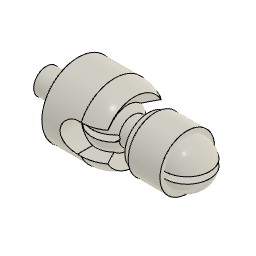
BallJoint2nd v2 (Autodesk Fusion 360 design; units mm, degrees)
Autodesk Fusion 360 part; units mm, degrees
sketch "スケッチ1" plane through (0, 0, 0) normal (0, 1, 0) x (1, 0, 0) in component "はめ込みジョイント"
  circle A0 centre (0, 0) radius 2.5
  line L0 (10, 1.5) -> (-2, 1.5)
  line L1 (-2, -1.5) -> (10, -1.5)
  line L2 (10, -1.5) -> (10, 1.5)
  line L3 (-2.5, 0) -> (10, 0)
  line L4 (1.7701, -0.35) -> (-2.4754, -0.35)
  line L5 (1.7701, 0.35) -> (-2.4754, 0.35)
  arc A1 (1.7701, -0.35) -> (1.7701, 0.35) centre (1.7701, 0) ccw
  dimension "d1" = 5
  dimension "d4" = 0.7
  constraint horizontal L0
  constraint parallel L0 L1
  constraint coincident A0.centre origin
  constraint midpoint L2 L3.end
  constraint coincident A0 L1.start
  constraint coincident A0 L3.start
  constraint coincident A0 L0.end
  constraint coincident L3 A1.centre
  constraint coincident A0 L4.end
  constraint tangent L4 A1
  constraint tangent L5 A1
  measures "d1" diameter of A0
  measures "d4" diameter of A1
revolve "回転1" add sketch "スケッチ1" angle 360 about axis through (-2.5, 0, 0) along (1, 0, 0) contours A0 L3 L4 A1 | A0 L1 L2 L3 | A0 L1 L3 L4 A1 | A0 L1 makes body 1 in component "はめ込みジョイント"
extrude "押し出し1" cut sketch "スケッチ1" along normal mid plane 6.2 contours A0 L3 L5 A1 | A0 L3 L4 A1 bodies 1 in component "はめ込みジョイント"
move_face "面を移動1" by (-6, 0, 0) 1 faces at (10, 0.5633, 0.8262) on bodies 1 in component "はめ込みジョイント"
mirror "ミラー1" about plane through (4, 0, 0) normal (1, 0, 0) of bodies 1 merged in component "はめ込みジョイント"
copy_body "ボディのコピーと貼り付け1" bodies 1 makes body 2 in component "はめ込みジョイント"
ref_plane "作業平面1" through (3, 0, 0) normal (1, 0, 0) x (0, 1, 0) in component "はめ込みジョイント"
split "分割1" by plane through (3, 0, 0) normal (1, 0, 0) bodies 2 makes body 3 at (7.9739, 2.1321, -1.3051) in component "はめ込みジョイント"
delete_body "RemoveBody1" bodies 3 in component "はめ込みジョイント"
ref_plane "作業平面2" through (4, 0, 0) normal (1, 0, 0) x (0, 1, 0) in component "はめ込みジョイント"
sketch "スケッチ2" plane through (4, 0, 0) normal (1, 0, 0) x (0, 1, 0) in component "はめ込みジョイント"
  circle A0 centre (0, 0) radius 3
  dimension "d12" = 6
  constraint coincident A0.centre origin
  measures "d12" diameter of A0
loft "ロフト1" add profiles "スケッチ2" section 1 face at (3, 0.5633, 0.8262) section 2 on bodies 2 bodies 2 in component "はめ込みジョイント"
extrude "押し出し2" add 1 faces at (4, -0.4661, 1.6472) along direction (1, 0, 0) blind 3 on bodies 2 bodies 2 in component "はめ込みジョイント"
sketch "スケッチ3" plane through (7, 0, 0) normal (1, 0, 0) x (0, 1, 0) in component "はめ込みジョイント"
  circle A0 centre (0, 0) radius 3
  circle A1 centre (0, 0) radius 1.6
  dimension "d15" = 3.2
  constraint concentric A0 A1
  measures "d15" diameter of A1
extrude "押し出し3" cut sketch "スケッチ3" against normal blind 3 contours A1 bodies 2 in component "はめ込みジョイント"
chamfer "面取り1" distance 0.5 angle 45 1 edges at (4, -2.797, 1.0848) on bodies 2 in component "はめ込みジョイント"
move_face "面を移動2" by (1, 0, 0) 1 faces at (7, -0.1889, 2.5207) on bodies 2 in component "はめ込みジョイント"
sketch "スケッチ4" plane through (0, 0, 0) normal (0, 1, 0) x (1, 0, 0) in component "はめ込みジョイント"
  circle A0 centre (0, 0) radius 2.6
  circle A1 centre (0, 0) radius 4
  line L0 (0, 0) -> (3, 0)
  line L1 (0, 0) -> (2.2021, -3.3393)
  line L2 (0, 0) -> (2.2021, 3.3393)
  line L3 (0, 0) -> (0, -0.2614)
  line L4 (0, -0.2614) -> (0, -4)
  line L5 (0, -4) -> (-4, -4)
  line L6 (-4, -4) -> (-4, 0)
  line L7 (-4, -4) -> (-8, -4)
  line L8 (-8, -4) -> (-8, 4)
  line L9 (-8, 4) -> (0, 4)
  line L10 (0, 0) -> (-8, 0)
  dimension "d19" = 5.2
  constraint coincident A0.centre A1.centre
  constraint coincident A1 L1.end
  constraint symmetric L0 A0.centre A1.centre
  constraint symmetric L0 L1.end L2.end
  constraint perpendicular L0 L3
  constraint coincident A1 L4.end
  constraint parallel L3 L4
  constraint tangent A1 L5
  constraint coincident A1 L6.end
  constraint tangent A1 L6
  constraint perpendicular L5 L6
  constraint perpendicular L6 L7
  constraint perpendicular L5 L8
  constraint coincident A1 L9.end
  constraint tangent A1 L9
  constraint perpendicular L8 L9
  constraint midpoint L8 L10.end
  measures "d19" diameter of A0
revolve "回転2" add sketch "スケッチ4" angle 360 about axis through (0, 0, 0) along (-1, 0, 0) separate body contours A0 A1 L1 L4 | A0 A1 L4 L10 | A1 L5 L6 | L6 L7 L8 L10 makes body 4 in component "はめ込みジョイント"
sketch "スケッチ5" plane through (0, 0, 0) normal (0, 1, 0) x (1, 0, 0) in component "はめ込みジョイント"
  circle A0 centre (-0.4, 0) radius 1.6
  line L0 (-0.4, 0) -> (-0.4, -1.6)
  line L1 (-0.4, 0) -> (-0.4, 1.6)
  line L2 (-0.4, -1.6) -> (4.9, -1.6)
  line L3 (4.9, -1.6) -> (4.9, 1.6)
  line L4 (4.9, 1.6) -> (-0.4, 1.6)
  dimension "d22" = 3.2
  constraint coincident A0.centre L0.start
  constraint vertical L0
  constraint coincident A0 L1.end
  constraint parallel L0 L1
  constraint perpendicular L0 L2
  constraint perpendicular L2 L3
  constraint perpendicular L1 L4
  measures "d22" diameter of A0
extrude "押し出し4" cut sketch "スケッチ5" along normal mid plane 9.2 bodies 4 in component "はめ込みジョイント"
sketch "スケッチ6" plane through (-8, 0, 0) normal (-1, 0, 0) x (0, -1, 0) in component "はめ込みジョイント"
  circle A0 centre (0, 0) radius 4
  circle A1 centre (0, 0) radius 1.6
  dimension "d25" = 3.2
  constraint coincident A0.centre A1.centre
  measures "d25" diameter of A1
extrude "押し出し5" cut sketch "スケッチ6" against normal blind 4 contours A1 bodies 4 in component "はめ込みジョイント"
copy_body "ボディのコピーと貼り付け2" bodies 4 makes body 5 in component "はめ込みジョイント"
extrude "押し出し6" cut 1 faces at (-8, -0.2386, 3.1836) along direction (1, 0, 0) blind 4 on bodies 5 bodies 5 in component "はめ込みジョイント"
move_face "面を移動3" by (0.5, 0, 0) 1 faces at (-4, 0.1832, -0.5939) on bodies 5 in component "はめ込みジョイント"
move_face "面を移動4" by (-0.5, 0, 0) 1 faces at (-3.5, 0.1832, -0.5939) on bodies 5 in component "はめ込みジョイント"
sketch "スケッチ7" plane through (-4, 0, 0) normal (-1, 0, 0) x (0, -1, 0) in component "はめ込みジョイント"
  circle A0 centre (0, 0) radius 4
  circle A1 centre (0, 0) radius 1.4
  dimension "d30" = 2.8
  constraint coincident A0.centre A1.centre
  measures "d30" diameter of A1
extrude "押し出し7" add sketch "スケッチ7" along normal blind 3.5 contours A1 bodies 5 in component "はめ込みジョイント"
component "はめ込みジョイント" placed x (1, 0, 0) y (0, 1, 0) z (0, 0, 1) at (0, 0, 0)
hidden bodies 4
named bodies: "B02", "B01", "B02 (1) (1)", "A01", "A02"
